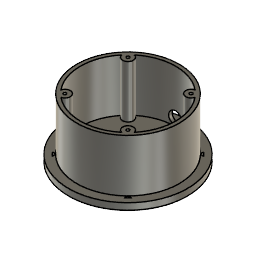
Base_J1 (Autodesk Fusion 360 design; units mm, degrees)
part number: 2026-07-09-14-32-38-014
Autodesk Fusion 360 part; units mm, degrees
sketch "スケッチ1" plane through (0, 0, 0) normal (0, 0, 1) x (1, 0, 0)
  line L0 (0, 0) -> (45, 0)
  line L1 (45, 0, 0) -> (45, 0, 6)
  line L2 (45, 0, 6) -> (40, 0, 6)
  line L3 (40, 0, 6) -> (40, 0, 50)
  line L4 (40, 0, 50) -> (37, 0, 50)
  line L5 (37, 0, 50) -> (37, 0, 6)
  line L6 (37, 0, 6) -> (0, 0, 6)
  line L7 (0, 0, 6) -> (0, 0, 0)
revolve "回転1" add sketch "スケッチ1" angle 360 about axis through (0, 0, 1.75) along (0, 0, 1) contours L0 L1 L2 L3 L4 L5 L6 L7 in plane through (0, 0, 0) normal (0, 1, 0)
sketch "スケッチ2" plane through (0, 0, 50) normal (0, 0, 1) x (1, 0, 0)
  circle A0 centre (0, 0) radius 40
  circle A1 centre (0, 0) radius 37
  line L0 (-20.25, -10) -> (20.25, -10)
  line L1 (20.25, -10) -> (20.25, 10)
  line L2 (20.25, 10) -> (-20.25, 10)
  line L3 (-20.25, 10) -> (-20.25, -10)
sketch "スケッチ3" plane through (0, 0, 0) normal (0, 0, 1) x (1, 0, 0)
  circle A0 centre (32.17, 32.17) radius 2.1
  circle A1 centre (-32.17, 32.17) radius 2.1
  circle A2 centre (-32.17, -32.17) radius 2.1
  circle A3 centre (32.17, -32.17) radius 2.1
extrude "押し出し2" cut sketch "スケッチ3" along normal blind 6 contours A0
extrude "押し出し3" cut sketch "スケッチ3" along normal blind 6 contours A2
extrude "押し出し4" cut sketch "スケッチ3" along normal blind 6 contours A1
extrude "押し出し5" cut sketch "スケッチ3" along normal blind 6 contours A3
sketch "スケッチ4" plane through (0, 0, 0) normal (0, 0, 1) x (1, 0, 0)
  circle A0 centre (33, 8.75) radius 1.8
  circle A1 centre (8, 8.75) radius 1.8
  circle A2 centre (8, -8.75) radius 1.8
  circle A3 centre (33, -8.75) radius 1.8
extrude "押し出し6" cut sketch "スケッチ4" along normal blind 6 contours A0
extrude "押し出し7" cut sketch "スケッチ4" along normal blind 6 contours A2
extrude "押し出し8" cut sketch "スケッチ4" along normal blind 6 contours A1
extrude "押し出し9" cut sketch "スケッチ4" along normal blind 6 contours A3
sketch "スケッチ6" plane through (0, 0, 0) normal (0, 0, 1) x (1, 0, 0)
  circle A0 centre (0, 0) radius 45
  circle A1 centre (0, 0) radius 48
extrude "FlangeWiden (1)" add sketch "スケッチ6" along normal blind 6
sketch "スケッチ7" plane through (0, 0, 0) normal (0, 0, 1) x (1, 0, 0)
  circle A0 centre (33, 8.75) radius 3.25
  circle A1 centre (8, 8.75) radius 3.25
  circle A2 centre (8, -8.75) radius 3.25
  circle A3 centre (33, -8.75) radius 3.25
extrude "ServoCounterbore (1)" cut sketch "スケッチ7" along normal blind 3
sketch "スケッチ8" plane through (0, 0, 0) normal (0, 1, 0) x (1, 0, 0)
  circle A0 centre (0, -12) radius 4
extrude "CableExit (1)" cut sketch "スケッチ8" along normal blind 45
fillet "FlangeRootFillet" radius 2 1 edges at (-37.2931, -14.4646, 6)
fillet "BoreFloorFillet" radius 0.5 1 edges at (-34.4961, -13.3798, 6)
sketch "スケッチ9" plane through (0, 0, 0) normal (0, 0, 1) x (1, 0, 0)
  circle A0 centre (0, 0) radius 48
  circle A1 centre (0, 0) radius 50
extrude "FlangeWiden2 (1)" add sketch "スケッチ9" along normal blind 6
chamfer "BottomChamfer" distance 0.5 angle 45 1 edges at (-46.6164, -18.0808, 0)
ref_plane "作業平面1" through (0, 0, 6) normal (0, 0, 1) x (1, 0, 0)
sketch "スケッチ10" plane through (0, 0, 6) normal (0, 0, 1) x (1, 0, 0)
  circle A0 centre (26.5, 26.5) radius 4.5
  circle A1 centre (-26.5, 26.5) radius 4.5
  circle A2 centre (-26.5, -26.5) radius 4.5
  circle A3 centre (26.5, -26.5) radius 4.5
extrude "PlateBosses (1)" add sketch "スケッチ10" along normal blind 44
ref_plane "作業平面2" through (0, 0, 50) normal (0, 0, 1) x (1, 0, 0)
sketch "スケッチ11" plane through (0, 0, 50) normal (0, 0, 1) x (1, 0, 0)
  circle A0 centre (26.5, 26.5) radius 1.25
  circle A1 centre (-26.5, 26.5) radius 1.25
  circle A2 centre (-26.5, -26.5) radius 1.25
  circle A3 centre (26.5, -26.5) radius 1.25
extrude "BossPilots (1)" cut sketch "スケッチ11" against normal blind 10
sketch "スケッチ12" plane through (0, 0, 6) normal (0, 0, 1) x (1, 0, 0)
  circle A0 centre (0, 0) radius 3.25
extrude "StubRelief (1)" cut sketch "スケッチ12" against normal blind 6
sketch "スケッチ13" plane through (0, 0, 0) normal (0, 0, 1) x (1, 0, 0)
sketch "スケッチ14" plane through (0, 0, 0) normal (0, 0, 1) x (1, 0, 0)
sketch "スケッチ15" plane through (0, 0, 0) normal (0, 1, 0) x (1, 0, 0)
  circle A0 centre (0, -12) radius 5.5
extrude "CableHoleBig (1)" cut sketch "スケッチ15" against normal blind 50
ref_plane "作業平面4" through (0, 0, 6) normal (0, 0, 1) x (1, 0, 0)
sketch "スケッチ16" plane through (0, 0, 6) normal (0, 0, 1) x (1, 0, 0)
  circle A0 centre (0, 0) radius 43
  circle A1 centre (0, 0) radius 40
extrude "WallThicken (1)" add sketch "スケッチ16" along normal blind 44
sketch "スケッチ17" plane through (0, 0, 6) normal (0, 0, 1) x (1, 0, 0)
  circle A0 centre (0, 0) radius 40
extrude "BoreEnlarge (1)" cut sketch "スケッチ17" along normal blind 44
sketch "スケッチ18" plane through (0, 0, 6) normal (0, 0, 1) x (1, 0, 0)
  circle A0 centre (26.5, 26.5) radius 4.5
  circle A1 centre (-26.5, 26.5) radius 4.5
  circle A2 centre (26.5, -26.5) radius 4.5
  circle A3 centre (-26.5, -26.5) radius 4.5
extrude "BossRestore (1)" add sketch "スケッチ18" along normal blind 44
ref_plane "作業平面5" through (0, 0, 40) normal (0, 0, 1) x (1, 0, 0)
sketch "スケッチ19" plane through (0, 0, 40) normal (0, 0, 1) x (1, 0, 0)
  circle A0 centre (26.5, 26.5) radius 1.25
  circle A1 centre (-26.5, 26.5) radius 1.25
  circle A2 centre (26.5, -26.5) radius 1.25
  circle A3 centre (-26.5, -26.5) radius 1.25
extrude "PilotRestore (1)" cut sketch "スケッチ19" along normal blind 10
sketch "スケッチ20" plane through (0, 0, 0) normal (0, 1, 0) x (1, 0, 0)
  circle A0 centre (0, -12) radius 5.5
extrude "CableHoleV2 (1)" cut sketch "スケッチ20" along normal blind 60
equation "d59 = -( 10.00 mm )"
equation "d116 = -( 6.00 mm )"
equation "d703 = -( 50.00 mm )"
